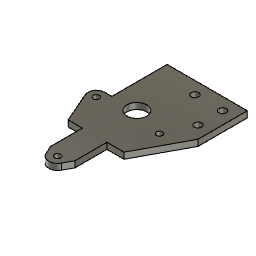
flasque roulement laser v3 (Autodesk Fusion 360 design; units mm, degrees)
Autodesk Fusion 360 part; units mm, degrees
sketch "Sketch1" plane through (0, 0, 0) normal (0, 0, 1) x (1, 0, 0)
  circle A0 centre (-25.7238, 28.3736) radius 2.5
  circle A1 centre (25.5, 28.3736) radius 2.5
  circle A2 centre (-0.0118, -28.6264) radius 2.5
  line L0 (45, 40) -> (45, 80)
  line L1 (45, 80) -> (25, 80)
  circle A3 centre (35, 50) radius 3
  circle A4 centre (12.5, 70) radius 3
  arc A5 (-6.6169, -31.6214) -> (6.3787, -32.0555) centre (-0.0118, -28.6264) ccw
  line L2 (-9.6692, 1.0232) -> (-9.6692, -24.8899)
  line L3 (10.2145, -24.9071) -> (10.2145, 1)
  line L4 (10.2145, 1) -> (24.0728, 1)
  line L5 (-9.6692, 1.0232) -> (-21.2251, 1.0232)
  line L6 (6.3787, -32.0555) -> (10.2145, -24.9071)
  line L7 (24.0728, 1) -> (45, 40)
  line L8 (-9.6692, -24.8899) -> (-6.6169, -31.6214)
  line L9 (-20, 35.1708) -> (-20, 80)
  line L10 (-20, 80) -> (25, 80)
  line L11 (-21.2251, 1.0232) -> (-31.7762, 25.2695)
  line L12 (-25.47, 35.1708) -> (-20, 35.1708)
  arc A6 (-25.47, 35.1708) -> (-31.7762, 25.2695) centre (-25.7238, 28.3736) ccw
  circle A7 centre (0, 35.5) radius 8
  circle A8 centre (35, 70) radius 3
  point P0 (0, 35.5)
  dimension "d43" = 16
  dimension "d46" = 6
  constraint vertical L0
  constraint horizontal L1
  constraint coincident A2.centre A5.centre
  constraint perpendicular L3 L4
  constraint perpendicular L2 L5
  constraint tangent A5 L6
  constraint parallel L6 L7
  constraint tangent A5 L8
  constraint perpendicular L9 L10
  constraint coincident A0.centre A6.centre
  constraint coincident P0 A7.centre
  measures "d43" diameter of A7
  measures "d46" diameter of A8
extrude "Extrude5" add sketch "Sketch1" along normal blind 5
